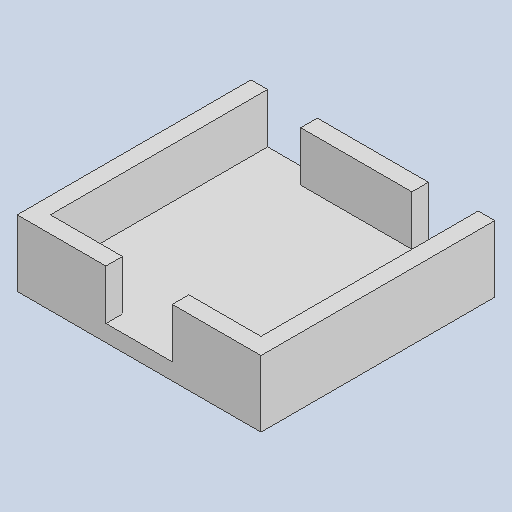
# Autodesk Inventor part: SMC-2000_case
Saved by Autodesk Inventor 2025.2 (Build 292293000, 293)
## iProperties
Created: 2025-07-30
Part Number: SMC-2000_case
Material: 일반
Document SubType Name: Modeling
Designer: jbhma
Density: 1 g/cm^3
Appearance: 기본값
Author: jbhma
Autodesk Inventor part; units mm, degrees
ref_plane "YZ Plane" through (0, 0, 0) normal (1, 0, 0) x (0, 1, 0)
ref_plane "XZ Plane" through (0, 0, 0) normal (0, 1, 0) x (-1, 0, 0)
ref_plane "XY Plane" through (0, 0, 0) normal (0, 0, 1) x (1, 0, 0)
sketch "스케치1" plane through (0, 0, 0) normal (0, 1, 0) x (-1, 0, 0)
  line L0 (36.75, -70.5) -> (-36.75, -70.5)
  line L1 (-36.75, -70.5) -> (-36.75, 0)
  line L2 (-36.75, 0) -> (36.75, 0)
  line L3 (36.75, 0) -> (36.75, -70.5)
  point P0 (0, 0)
  point P1 (0, 0)
  dimension "d0" = 70.5
  dimension "d1" = 73.5
  constraints: 8 end point, 2 parallel, 1 coincident, 1 horizontal, 1 midpoint, 1 perpendicular
  measures "d0" distance between parallel lines of L0 L2
  measures "d1" distance between parallel lines of L1 L3
extrude "돌출1" add sketch "스케치1" along normal blind 5
sketch "스케치2" plane through (0, 5, 0) normal (0, 1, 0) x (1, 0, 0)
  line L0 (-36.75, 0) -> (36.75, 0) projected
  line L1 (36.75, 0) -> (36.75, 70.5) projected
  line L2 (36.75, 70.5) -> (-36.75, 70.5) projected
  line L3 (-36.75, 70.5) -> (-36.75, 0) projected
  line L4 (-36.75, 70.5) -> (36.75, 70.5)
  line L5 (36.75, 70.5) -> (36.75, 0)
  line L6 (36.75, 0) -> (-36.75, 0)
  line L7 (-36.75, 0) -> (-36.75, 70.5)
  line L8 (-31.75, 65.5) -> (31.75, 65.5)
  line L9 (31.75, 65.5) -> (31.75, 5)
  line L10 (31.75, 5) -> (-31.75, 5)
  line L11 (-31.75, 5) -> (-31.75, 65.5)
  point P0 (0, 0)
  dimension "d4" = 5
  constraints: 16 end point, 2 parallel, 1 horizontal, 1 perpendicular, 3 other
  measures "d4" distance between parallel lines of L2 L8
extrude "돌출2" add sketch "스케치2" along normal blind 15
sketch "스케치3" plane through (-36.75, 0, 0) normal (0, 0, 1) x (1, 0, 0)
  line L0 (0, 0) -> (73.5, 0) projected
  line L1 (73.5, 0) -> (73.5, 20) projected
  line L2 (0, 20) -> (73.5, 20) projected
  line L3 (0, 0) -> (0, 20) projected
  line L4 (26.75, 20) -> (46.75, 20)
  line L5 (46.75, 20) -> (46.75, 5)
  line L6 (46.75, 5) -> (26.75, 5)
  line L7 (26.75, 5) -> (26.75, 20)
  point P0 (36.75, 0)
  point P1 (36.75, 20)
  dimension "d7" = 20
  dimension "d8" = 15
  constraints: 8 end point, 2 midpoint, 2 parallel, 1 horizontal, 1 perpendicular, 1 point on line
  measures "d7" distance of L5.end L6.end
  measures "d8" distance of L4.end L5.end
extrude "돌출3" cut sketch "스케치3" against normal blind 15 contours L2 L5 L6 L7
sketch "스케치4" plane through (36.75, 0, -70.5) normal (0, 0, -1) x (-1, 0, 0)
  line L0 (0, 0) -> (73.5, 0) projected
  line L1 (73.5, 0) -> (73.5, 20) projected
  line L2 (0, 20) -> (73.5, 20) projected
  line L3 (0, 0) -> (0, 20) projected
  line L4 (5, 20) -> (20, 20)
  line L5 (20, 20) -> (20, 5)
  line L6 (20, 5) -> (5, 5)
  line L7 (5, 5) -> (5, 20)
  line L8 (53.5, 20) -> (68.5, 20)
  line L9 (68.5, 20) -> (68.5, 5)
  line L10 (68.5, 5) -> (53.5, 5)
  line L11 (53.5, 5) -> (53.5, 20)
  point P0 (36.75, 0)
  point P1 (20, 20)
  dimension "d11" = 15
  dimension "d12" = 15
  dimension "d13" = 15
  dimension "d14" = 15
  dimension "d15" = 5
  dimension "d16" = 5
  constraints: 16 end point, 4 parallel, 2 horizontal, 2 perpendicular, 2 point on line
  measures "d11" distance of L5.end L6.end
  measures "d12" distance of L4.end L5.end
  measures "d13" distance of L9.end L10.end
  measures "d14" distance of L8.end L9.end
  measures "d15" distance between parallel lines of L3 L7
  measures "d16" distance between parallel lines of L1 L9
extrude "돌출4" cut sketch "스케치4" against normal blind 5 contours L2 L5 L6 L7 | L9 L10 L11 L2
